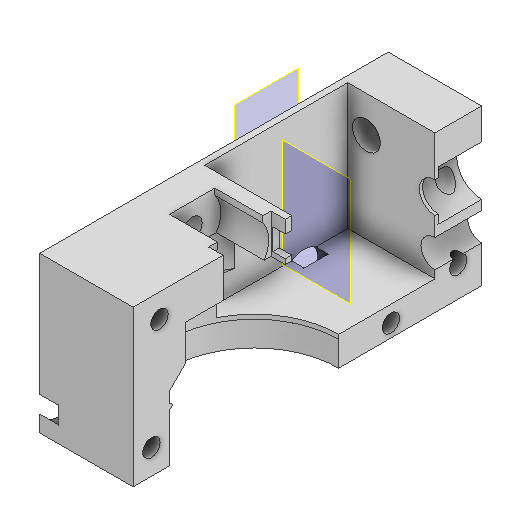
# Autodesk Inventor part: 10_SOOCT_Base_v1
Saved by Autodesk Inventor 2022 (Build 260153000, 153)
## iProperties
Created: 2023-01-02
Part Number: 10_SOOCT_Base_v1
Material: Generisch
Document SubType Name: Modeling
Designer: diederichbenedict
Density: 1 g/cm^3
Appearance: Vorgabe
Author: diederichbenedict
Autodesk Inventor part; units mm, degrees
ref_plane "YZ Plane" through (0, 0, 0) normal (1, 0, 0) x (0, 1, 0)
ref_plane "Arbeitsebene1" through (-39.7131, -1.3218, -40.6417) normal (-1, 0, 0) x (0, 0, -1)
sketch "Skizze1" plane through (-39.7131, -1.3218, -40.6417) normal (-1, 0, 0) x (0, 0, -1)
  line L0 (-10.1, 42.0592) -> (-10.1, 20.2092)
  line L1 (-10.1, 19.2092) -> (-10.1, 18.0592)
  line L2 (-37.1, 42.0592) -> (-37.1, 20.2092)
  line L3 (-37.1, 19.2092) -> (-37.1, 18.0592)
  line L4 (4, 5) -> (1, 5)
  line L5 (-37.1, 27.2) -> (-43.1, 27.2)
  line L6 (-43.1, 27.2) -> (-43.1, 3.2)
  line L7 (-43.1, 3.2) -> (-37.1, 3.2)
  line L8 (-37.1, 3.2) -> (-37.1, 27.2)
  line L9 (-7.8, 3.2) -> (0, 3.2)
  line L10 (-37.1, 3.2) -> (12.9, 3.2)
  line L11 (12.9, 3.2) -> (12.9, 27.2)
  line L12 (12.9, 27.2) -> (-37.1, 27.2)
  line L13 (-37.1, 27.2) -> (-37.1, 3.2)
  point P0 (-40.6417, -1.3218)
  point P1 (-37.1, 24.2092)
  point P2 (-7.8, 3.2)
  dimension "d0" = 0
  dimension "d2" = 6
  dimension "d3" = 50
  dimension "d21" = 24
  constraints: 28 end point, 4 horizontal, 4 parallel, 4 vertical, 2 perpendicular, 1 point on line, 12 other
  measures "d0" distance between parallel lines of L7 L9
  measures "d2" distance between parallel lines of L8 L6
  measures "d3" distance of L5.start L11.end
  measures "d21" distance between parallel lines of L12 L7
extrude "Extrusion1" add sketch "Skizze1" against normal up to surface (17 mm away)
sketch "Skizze2" plane through (-22.7131, -28.5218, 2.4583) normal (1, 0, 0) x (0, 0, -1)
  line L0 (33, 5) -> (33, 6.15)
  line L1 (33, -17.85) -> (33, 4)
  line L2 (0, 24) -> (56, 24)
  line L3 (8.5007, 24) -> (8.5007, 12.0658)
  line L4 (8.5007, 12.0658) -> (5.9, 9.4651)
  line L5 (5.9, 9.4651) -> (5.9, 7.6275)
  arc A0 (5.9, 6.8275) -> (5.9, 7.6275) centre (5.9, 7.2275) ccw
  line L6 (5.9, 6.8275) -> (5.9, -14.594)
  line L7 (56.2565, 0) -> (0.3327, 0)
  line L8 (15.7023, 20.4) -> (24.9625, 20.4029)
  line L9 (19.4614, 24) -> (19.4689, 0)
  line L10 (33, 7.9908) -> (6, 7.9908) projected
  line L11 (33, 6.9908) -> (6, 6.9908) projected
  line L12 (56, 24) -> (0, 24) projected
  line L13 (6, 7.9908) -> (6, 9.1408)
  line L14 (56, 0) -> (56, 24) projected
  line L15 (56, 24) -> (0, 24) projected
  line L16 (0, 24) -> (0, 0) projected
  line L17 (0, 0) -> (56, 0) projected
  line L18 (6, 9.1408) -> (14, 17.1408)
  point P0 (2.4583, 28.5218)
  point P1 (5.9, 0)
  point P2 (7.3142, 24)
  dimension "d10" = 5.5
  dimension "d37" = 0
  dimension "d38" = 0.1
  dimension "d39" = 0
  dimension "d40" = 0.8
  dimension "d41" = 0.3
  constraints: 24 end point, 6 point on line, 2 collinear, 2 parallel, 2 point on circle, 1 centre point, 1 coincident, 1 vertical, 3 other
  measures "d10" distance from line of L8.end L9
  measures "d37" distance between parallel lines of L12 L2
  measures "d38" distance between parallel lines of L13 L5
  measures "d39" distance between parallel lines of L6 L5
  measures "d40" distance of L5.end L6.start
  measures "d41" distance between parallel lines of L18 L4
revolve "Umdrehung1" cut sketch "Skizze2" angle 360 about axis through (-22.7131, -4.5218, -17.0031) along (0, -1, -0.0003154) contours L2 L9 L11 A0 L5 L4 L3 | L6 A0 L11 L9 L7
sketch "Skizze3" plane through (-22.7131, -28.5218, -53.5417) normal (1, 0, 0) x (0, 0, -1)
  line L0 (-38.5, 18.2) -> (-38.5, 22.2) projected
  line L1 (-34.5, 18.2) -> (-38.5, 18.2) projected
  line L2 (-34.5, 22.2) -> (-34.5, 18.2) projected
  line L3 (-38.5, 22.2) -> (-34.5, 22.2) projected
  line L4 (-34, 22.7) -> (-34, 17.7)
  line L5 (-34, 17.7) -> (-39, 17.7)
  line L6 (-39, 17.7) -> (-39, 22.7)
  line L7 (-39, 22.7) -> (-34, 22.7)
  line L8 (-47.4993, 12.0658) -> (-47.4993, 24) projected
  line L9 (-25.578, 24) -> (-25.5704, 12.0727) projected
  line L10 (-47.4993, 22.7) -> (-25.574, 22.7)
  line L11 (-25.574, 22.7) -> (-25.574, 17.7)
  line L12 (-25.574, 17.7) -> (-47.4993, 17.7)
  line L13 (-47.4993, 17.7) -> (-47.4993, 22.7)
  line L14 (-47.4993, 22.7) -> (-25.578, 22.7)
  line L15 (-25.578, 22.7) -> (-25.578, 24)
  line L16 (-25.578, 24) -> (-47.4993, 24)
  line L17 (-47.4993, 24) -> (-47.4993, 22.7)
  point P0 (-53.5417, 28.5218)
  point P1 (-47.4993, 17.7)
  point P2 (-34, 14.7092)
  point P3 (-25.5771, 22.7)
  point P4 (-34, 19.7092)
  point P5 (-34, 19.7092)
  point P6 (-34, 22.7)
  point P7 (-34, 17.7)
  point P8 (-47.4993, 24)
  point P9 (-25.578, 22.7)
  dimension "d12" = 0.5
  constraints: 24 end point, 4 parallel, 4 point on line, 2 horizontal, 2 perpendicular, 3 other
  measures "d12" distance between parallel lines of L3 L7
extrude "Extrusion2" add sketch "Skizze3" against normal through all contours L0 L3 L2 L1 | L10 L9 L12 L4 | L4 L5 L6 L7 | L7 L10 L8 L16 L9 | L6 L12 L8 L10 | L10 L11 L9
sketch "Skizze4" plane through (-22.7131, -28.5218, -53.5417) normal (1, 0, 0) x (0, 0, -1)
  line L0 (-38.5, 18.2) -> (-38.5, 22.2) projected
  line L1 (-34.5, 18.2) -> (-38.5, 18.2) projected
  line L2 (-34.5, 22.2) -> (-34.5, 18.2) projected
  line L3 (-38.5, 22.2) -> (-34.5, 22.2) projected
  line L4 (-34.45, 22.25) -> (-34.45, 18.15)
  line L5 (-34.45, 18.15) -> (-38.55, 18.15)
  line L6 (-38.55, 18.15) -> (-38.55, 22.25)
  line L7 (-38.55, 22.25) -> (-34.45, 22.25)
  line L8 (-56, 0) -> (-50.1, 0) projected
  line L9 (0, 0) -> (0, 24) projected
  line L10 (0, 24) -> (-25.578, 24) projected
  line L11 (-56, 24) -> (-56, 0) projected
  line L12 (-38.2, 22.25) -> (-34.8, 22.25)
  line L13 (-34.8, 22.25) -> (-34.8, 22.7)
  line L14 (-34.8, 22.7) -> (-38.2, 22.7)
  line L15 (-38.2, 22.7) -> (-38.2, 22.25)
  line L16 (-34.5, 18.2) -> (-34.5, 22.2)
  line L17 (-38.25, 18.15) -> (-34.75, 18.15)
  line L18 (-34.75, 18.15) -> (-34.75, 17.7)
  line L19 (-34.75, 17.7) -> (-38.25, 17.7)
  line L20 (-38.25, 17.7) -> (-38.25, 18.15)
  line L21 (-25.578, 24) -> (-25.5771, 22.7) projected
  line L22 (-25.5704, 12.0727) -> (-22.9681, 9.4737) projected
  line L23 (-22.9681, 9.4737) -> (-22.9669, 7.6361) projected
  arc A0 (-22.9669, 7.6361) -> (-22.9664, 6.8361) centre (-22.9667, 7.2361) ccw projected
  line L24 (-22.9664, 6.8361) -> (-22.9621, 0.0086) projected
  line L25 (-47.4993, 12.0658) -> (-47.4993, 17.7) projected
  line L26 (-50.1, 0) -> (-50.1, 6.8275) projected
  arc A1 (-50.1, 6.8275) -> (-50.1, 7.6275) centre (-50.1, 7.2275) ccw projected
  line L27 (-50.1, 7.6275) -> (-50.1, 9.4651) projected
  line L28 (-50.1, 9.4651) -> (-47.4993, 12.0658) projected
  line L29 (-47.4993, 17.7) -> (-25.574, 17.7) projected
  line L30 (-25.574, 17.7) -> (-25.5704, 12.0727) projected
  line L31 (-25.5771, 22.7) -> (-25.578, 22.7) projected
  line L32 (-22.9621, 0.0086) -> (-36.5311, 0) projected
  line L33 (-36.5311, 0) -> (0, 0) projected
  line L34 (-25.578, 22.7) -> (-25.578, 24) projected
  line L35 (-25.578, 24) -> (-56, 24) projected
  line L36 (-38.2, 22.7) -> (-34.8, 22.7)
  line L37 (-34.8, 22.7) -> (-34.8, 24)
  line L38 (-34.8, 24) -> (-38.2, 24)
  line L39 (-38.2, 24) -> (-38.2, 22.7)
  line L40 (-34.45, 21.95) -> (-21.9312, 21.95)
  line L41 (-21.9312, 21.95) -> (-21.9312, 18.5)
  line L42 (-21.9312, 18.5) -> (-34.45, 18.5)
  line L43 (-34.45, 18.5) -> (-34.45, 21.95)
  point P0 (-53.5417, 28.5218)
  point P1 (-43.6858, 14.7092)
  point P2 (-19.3142, 14.7092)
  point P3 (-47.4993, 22.7)
  point P4 (-34.75, 18.15)
  point P5 (-34.8059, 22.7)
  point P6 (-34.45, 18.5)
  dimension "d15" = 0.05
  dimension "d58" = 0.3
  dimension "d59" = 0.3
  dimension "d60" = 0.3
  dimension "d61" = 0.3
  dimension "d64" = 0.3
  dimension "d65" = 0.3
  constraints: 42 end point, 8 parallel, 5 point on line, 4 horizontal, 4 perpendicular, 3 other
  measures "d15" distance between parallel lines of L3 L7
  measures "d58" distance between parallel lines of L0 L15
  measures "d59" distance between parallel lines of L2 L37
  measures "d60" distance between parallel lines of L4 L18
  measures "d61" distance between parallel lines of L20 L6
  measures "d64" distance between parallel lines of L7 L40
  measures "d65" distance between parallel lines of L42 L1
extrude "Extrusion3" cut sketch "Skizze4" against normal blind 2 contours L0 L3 L2 L1 | L4 L5 L6 L7 | L40 L41 L42 L4 | L7 L15 L14 L13 | L14 L39 L35 L37 | L18 L19 L20 L5
sketch "Skizze5" plane through (-39.7131, -28.5218, -53.5417) normal (0, 0, -1) x (-1, 0, 0)
  arc A0 (-8, 26.2) -> (-9, 27.2) centre (-9, 26.2) ccw projected
  line L0 (-25, 27.2) -> (-9, 27.2) projected
  arc A1 (-25, 27.2) -> (-26, 26.2) centre (-25, 26.2) ccw projected
  line L1 (-26, 10.2) -> (-26, 26.2) projected
  arc A2 (-26, 10.2) -> (-25, 9.2) centre (-25, 10.2) ccw projected
  line L2 (-9, 9.2) -> (-25, 9.2) projected
  arc A3 (-9, 9.2) -> (-8, 10.2) centre (-9, 10.2) ccw projected
  line L3 (-8, 26.2) -> (-8, 10.2) projected
  circle A4 centre (-17, 18.2) radius 5.8 projected
  arc A5 (-9, 8.2) -> (-7, 10.2) centre (-9, 10.2) ccw
  line L4 (-9, 8.2) -> (-25, 8.2)
  arc A6 (-27, 10.2) -> (-25, 8.2) centre (-25, 10.2) ccw
  line L5 (-27, 10.2) -> (-27, 26.2)
  arc A7 (-25, 28.2) -> (-27, 26.2) centre (-25, 26.2) ccw
  line L6 (-25, 28.2) -> (-9, 28.2)
  arc A8 (-7, 26.2) -> (-9, 28.2) centre (-9, 26.2) ccw
  line L7 (-7, 26.2) -> (-7, 10.2)
  line L8 (-31, 32.2) -> (-3, 32.2)
  line L9 (-3, 32.2) -> (-3, 4.2)
  line L10 (-3, 4.2) -> (-31, 4.2)
  line L11 (-31, 4.2) -> (-31, 32.2)
  line L12 (-31, 32.2) -> (-3, 4.2) construction
  line L13 (-3, 32.2) -> (-31, 4.2) construction
  point P0 (-39.7131, 28.5218)
  dimension "d18" = 1
  dimension "d27" = 28
  dimension "d28" = 28
  constraints: 20 end point, 8 point on circle, 4 centre point, 2 midpoint, 2 parallel, 1 horizontal, 1 perpendicular, 7 other
  measures "d18" distance between parallel lines of L3 L7
  measures "d27" distance of L9.end L10.end
  measures "d28" distance of L8.end L9.end
extrude "Extrusion4" cut sketch "Skizze5" against normal blind 23.5 contours L3 A3 L2 A2 L1 A1 L0 A0 | A4 | L4 A6 L5 A7 L6 A8 L7 A5
sketch "Skizze6" plane through (-39.7131, -28.5218, -53.5417) normal (0, 0, -1) x (-1, 0, 0)
  line L0 (-9, 8.2) -> (-17, 8.2) projected
  line L1 (-17, 0) -> (-17, 8.2) projected
  line L2 (0, 0) -> (-17, 0) projected
  line L3 (0, 24) -> (0, 0) projected
  line L4 (0, 24) -> (-7, 24) projected
  line L5 (-7, 24) -> (-7, 10.2) projected
  arc A0 (-9, 8.2) -> (-7, 10.2) centre (-9, 10.2) ccw projected
  line L6 (-17, 8.2) -> (-17, 12.0727) projected
  line L7 (-17, 8.2) -> (-7, 8.2)
  line L8 (-7, 8.2) -> (-7, 24)
  line L9 (-7, 24) -> (-17, 24)
  line L10 (-17, 24) -> (-17, 8.2)
  circle A1 centre (-17, 18.2) radius 4 projected
  circle A2 centre (-17, 15.0113) radius 4
  point P0 (-39.7131, 28.5218)
  point P1 (-17, 22.2)
  point P2 (-17, 14.2)
  point P3 (-17, 19.0113)
  point P4 (-17, 11.0113)
  constraints: 8 end point, 2 parallel, 1 centre point, 1 horizontal, 1 perpendicular, 2 other
ref_plane "Arbeitsebene2" through (-26.7131, -14.3218, -41.6417) normal (0, 0, 1) x (1, 0, 0)
ref_plane "Arbeitsebene3" through (-26.7131, -14.3218, -44.6417) normal (0, 0, -1) x (0, 1, 0)
extrude "Extrusion5" add sketch "Skizze6" against normal blind 8 contours L0 L6 A2 A1 L10 L9 L5 A0 | A1 A2 L10 picked at (-16.3965, 20.005)
sketch "Skizze7" plane through (-32.7131, -4.5218, -45.5417) normal (0, 0, 1) x (1, 0, 0)
  circle A0 centre (10, -5.8) radius 4
  line L0 (10, 0) -> (10, -24) projected
  line L1 (10, -9.8) -> (10, -1.8)
  circle A1 centre (10, -5.8) radius 3
  circle A2 centre (10, -8.9887) radius 4 projected
  point P0 (32.7131, 4.5218)
  point P1 (10, -8.8)
  point P2 (10, -2.8)
  dimension "d24" = 1
  constraints: 2 centre point, 2 end point, 1 point on circle
  measures "d24" radial gap between concentric circles of A0 A1
extrude "Extrusion6" add sketch "Skizze7" against normal blind 0.5 contours L0 A1 A2 A0 | A2 A1 L0 A0 picked at (9.6732, -2.174) picked at (9.6932, -9.4309)
ref_plane "Arbeitsebene4" through (-39.7131, -28.5218, -32.0417) normal (0, 0, -1) x (-1, 0, 0)
sketch "Skizze8" plane through (-39.7131, -28.5218, -32.0417) normal (0, 0, -1) x (-1, 0, 0)
  circle A0 centre (-17, 18.2) radius 4 projected
  line L0 (-3, 3.7) -> (-31, 3.7)
  line L1 (-31, 3.7) -> (-31, 32.7)
  line L2 (-31, 32.7) -> (-3, 32.7)
  line L3 (-3, 32.7) -> (-3, 3.7)
  line L4 (-17, 22.2) -> (-17, 18.2) projected
  line L5 (-3, 3.7) -> (-31, 32.7) construction
  line L6 (-31, 3.7) -> (-3, 32.7) construction
  point P0 (-39.7131, 28.5218)
  dimension "d30" = 28
  dimension "d31" = 29
  constraints: 12 end point, 2 midpoint, 2 parallel, 1 horizontal, 1 perpendicular, 1 vertical alignment
  measures "d30" distance of L1.end L2.end
  measures "d31" distance of L0.end L1.end
extrude "Extrusion7" cut sketch "Skizze8" along normal blind 14 and the other way blind 9 contours A0 | L0 L1 L2 L3
sketch "Skizze9" plane through (-39.7131, -28.5218, -53.5417) normal (0, 0, -1) x (-1, 0, 0)
  circle A0 centre (-17, 7.2) radius 2.2504 projected
  circle A1 centre (-6, 18.2) radius 2.2504 projected
  point P0 (-39.7131, 28.5218)
extrude "Extrusion8" cut sketch "Skizze9" against normal blind 14
sketch "Skizze10" plane through (-39.7131, -28.5218, -53.5417) normal (0, -1, 0) x (1, 0, 0)
  line L0 (8.5019, 6.0924) -> (3.4981, 6.0924) projected
  line L1 (17, 56) -> (17, 50.1) projected
  line L2 (0, 56) -> (17, 56) projected
  line L3 (0, 0) -> (0, 56) projected
  line L4 (0, 0) -> (17, 0) projected
  line L5 (17, 36.5311) -> (17, 0) projected
  line L6 (17, 50.1) -> (17, 36.5311) projected
  ellipse E0 centre (17, 36.5311) end of major axis (30.5689, 36.5311) minor radius 13.5689 (17, 50.1) -> (17, 22.9621) ccw projected
  point P0 (39.7131, 53.5417)
  constraints: 1 other
extrude "Extrusion9" cut sketch "Skizze10" against normal blind 3 contours L6 L5 E0
sketch "Skizze11" plane through (-39.7131, -28.5218, -53.5417) normal (0, -1, 0) x (1, 0, 0)
  circle A0 centre (17, 36.5) radius 13.5 projected
  ellipse E0 centre (17, 36.5311) end of major axis (30.5689, 36.5311) minor radius 13.5689 (17, 50.1) -> (17, 22.9621) ccw projected
  line L0 (17, 56) -> (17, 50.1) projected
  line L1 (0, 56) -> (17, 56) projected
  line L2 (0, 0) -> (0, 56) projected
  line L3 (0, 0) -> (17, 0) projected
  line L4 (17, 22.9621) -> (17, 0) projected
  point P0 (39.7131, 53.5417)
  constraints: 1 other
extrude "Extrusion10" add sketch "Skizze11" along normal blind 3 contours E0 L4 L3 L2 L1 L0
sketch "Skizze12" plane through (-39.7131, -1.3218, -40.6417) normal (-1, 0, 0) x (0, 0, 1)
  circle A0 centre (40.15, -24.2) radius 1.29
  circle A1 centre (38.86, -7) radius 1.4
  circle A2 centre (-9.15, -23.4127) radius 1.4
  circle A3 centre (1.6677, -26.1156) radius 1.4
  circle A4 centre (-10.55, -14.0018) radius 1.4
  line L0 (-12.9, -11.2504) -> (-5.4, -11.2504) projected
  line L1 (-12.9, -22.2504) -> (-5.4, -22.2504) projected
  line L2 (-12.9, -6.7496) -> (-5.4, -6.7496) projected
  point P0 (40.6417, 1.3218)
  dimension "d46" = 2.58
  dimension "d47" = 2.8
  dimension "d48" = 2.8
  dimension "d49" = 2.8
  dimension "d50" = 2.8
  constraints: 5 centre point
  measures "d46" diameter of A0
  measures "d47" diameter of A1
  measures "d48" diameter of A2
  measures "d49" diameter of A3
  measures "d50" diameter of A4
hole "Bohrung1" at (-39.7131, -25.5218, -0.4917) at (-39.7131, -8.3218, -1.7817) at (-39.7131, -27.4374, -38.974) at (-39.7131, -24.7346, -49.7917) at (-39.7131, -15.3236, -51.1917) direction (1, 0, 0) diameter 2.8 end through all counterbore diameter 6.5 counterbore depth 5
sketch "Skizze13" plane through (-39.7131, -1.3218, -40.6417) normal (-1, 0, 0) x (0, 0, 1)
  line L0 (37.2, -30.2) -> (43.1, -30.2) projected
  line L1 (43.1, -30.2) -> (-14.489, -30.2)
  line L2 (-14.489, -30.2) -> (-14.489, -1.9274)
  line L3 (-14.489, -1.9274) -> (43.1, -1.9274)
  line L4 (43.1, -1.9274) -> (43.1, -30.2)
  point P0 (40.6417, 1.3218)
  point P1 (37.2, -30.2)
  constraints: 8 end point, 2 parallel, 1 horizontal, 1 perpendicular
extrude "Extrusion11" cut sketch "Skizze13" against normal blind 2
sketch "Skizze14" plane through (-39.7131, -28.5218, -46.0417) normal (0, 0, 1) x (1, 0, 0)
  arc A0 (17, 19.0113) -> (17, 11.0113) centre (17, 15.0113) ccw projected
  circle A1 centre (17, 15.0113) radius 2.5
  line L0 (17, 11.0113) -> (17, 9.4504) projected
  line L1 (17, 11.0113) -> (17, 19.0113)
  point P0 (39.7131, 28.5218)
  point P1 (17, 12.5113)
  point P2 (17, 17.5113)
  dimension "d68" = 5
  constraints: 2 end point, 1 centre point, 1 coincident, 1 collinear
  measures "d68" diameter of A1
extrude "Extrusion12" add sketch "Skizze14" against normal blind 0.5 contours L1 A1 A0
sketch "Skizze15" plane through (-37.7131, -1.3218, -40.6417) normal (-1, 0, 0) x (0, 0, 1)
  circle A0 centre (1.6677, -26.1156) radius 3.25 projected
  circle A1 centre (38.86, -7) radius 3.25 projected
  circle A2 centre (-9.15, -23.4127) radius 3.25 projected
  arc A3 (43.1, -22.8362) -> (43.1, -25.5638) centre (40.15, -24.2) ccw projected
  line L0 (43.1, -3.2) -> (43.1, -22.8362) projected
  line L1 (-12.9, -3.2) -> (43.1, -3.2) projected
  line L2 (-12.9, -11.7568) -> (-12.9, -3.2) projected
  arc A4 (-12.9, -16.2468) -> (-12.9, -11.7568) centre (-10.55, -14.0018) ccw projected
  line L3 (-12.9, -30.2) -> (-12.9, -16.2468) projected
  line L4 (43.1, -30.2) -> (-12.9, -30.2) projected
  line L5 (43.1, -25.5638) -> (43.1, -30.2) projected
  line L6 (43.1, -3.2) -> (43.1, -30.2) projected
  line L7 (-12.9, -30.2) -> (43.1, -30.2)
  line L8 (43.1, -30.2) -> (43.1, -28.2)
  line L9 (43.1, -28.2) -> (-12.9, -28.2)
  line L10 (-12.9, -28.2) -> (-12.9, -30.2)
  point P0 (40.6417, 1.3218)
  dimension "d71" = 2
  constraints: 8 end point, 2 parallel, 1 horizontal, 1 perpendicular, 1 point on line
  measures "d71" distance of L8.end L7.end
extrude "Extrusion13" cut sketch "Skizze15" against normal through all contours L9 A0 | A0 L9 L5 L4 L3 picked at (1.0341, -28.384)
sketch "Skizze16" plane through (-22.7131, -20.8943, -3.4417) normal (1, 0, 0) x (0, 0, -1)
  circle A0 centre (13.6, 12.5725) radius 4.6
  line L0 (50.1, 16.3725) -> (-5.9, 16.3725) projected
  line L1 (9.9503, 16.3725) -> (9.9503, 15.3725)
  line L2 (9.9503, 16.3725) -> (10.9503, 16.3725) construction
  line L3 (17.2497, 16.3725) -> (17.2497, 15.3725)
  line L4 (11.55, 14.6225) -> (15.65, 10.5225)
  line L5 (15.65, 10.5225) -> (15.65, 14.6225)
  line L6 (15.65, 14.6225) -> (11.55, 10.5225)
  point P0 (-3.4417, 20.8943)
  point P1 (16.1923, 16.3725)
  point P2 (11.0077, 16.3725)
  dimension "d74" = 9.2
  dimension "d80" = 90
  dimension "d81" = 1
  dimension "d82" = 1
  constraints: 12 end point, 3 midpoint, 2 perpendicular, 2 point on circle, 2 point on line, 2 vertical, 1 centre point, 1 horizontal
  measures "d74" diameter of A0
  measures "d80" angle of L1 L2
  measures "d81" distance of L1.end L1.start
  measures "d82" distance from line of L3.end L0
extrude "Extrusion14" cut sketch "Skizze16" against normal blind 10 contours A0 L0 | A0 L0 L3 | L1 L0 A0 | L0 A0 | L6 L5 L4
sketch "Skizze18" plane through (-22.7131, -20.8943, -3.4417) normal (1, 0, 0) x (0, 0, -1)
  line L0 (9.9503, 15.3725) -> (9.9503, 16.3725) projected
  line L1 (9.9503, 16.3725) -> (-5.9, 16.3725) projected
  line L2 (-5.9, 16.3725) -> (-5.9, -8.6275) projected
  line L3 (-5.9, -8.6275) -> (0, -8.6275) projected
  line L4 (0, -4.6275) -> (0, -8.6275) projected
  line L5 (0, -4.6275) -> (0, -0.8) projected
  arc A0 (0, -0.8) -> (0, 0) centre (0, -0.4) ccw projected
  line L6 (0, 0) -> (0, 1.8376) projected
  line L7 (0, 1.8376) -> (2.6007, 4.4383) projected
  line L8 (2.6007, 4.4383) -> (2.6007, 10.0725) projected
  line L9 (2.6007, 10.0725) -> (9.7387, 10.0725) projected
  arc A1 (9.9503, 15.3725) -> (9.7387, 10.0725) centre (13.6, 12.5725) ccw projected
  circle A2 centre (-2.95, -4.6275) radius 1.4 projected
  circle A3 centre (-1.66, 12.5725) radius 1.4 projected
  arc A4 (8.9719, 11.9725) -> (10.3013, 10.0882) centre (10.9719, 11.9725) ccw projected
  arc A5 (11.9719, 16.3512) -> (10.3013, 10.0882) centre (13.5632, 12.5725) ccw projected
  line L10 (11.9719, 16.6725) -> (11.9719, 16.3512) projected
  line L11 (8.9719, 16.6725) -> (11.9719, 16.6725) projected
  line L12 (8.9719, 11.9725) -> (8.9719, 16.6725) projected
  line L13 (18.5632, 7.5725) -> (8.5632, 7.5725)
  line L14 (8.5632, 7.5725) -> (8.5632, 17.5725)
  line L15 (8.5632, 17.5725) -> (18.5632, 17.5725)
  line L16 (18.5632, 17.5725) -> (18.5632, 7.5725)
  line L17 (18.5632, 7.5725) -> (8.5632, 17.5725) construction
  line L18 (8.5632, 7.5725) -> (18.5632, 17.5725) construction
  point P0 (-3.4417, 20.8943)
  point P1 (9.36, 10.7885)
  point P2 (8.5632, 10.0725)
  point P3 (8.5632, 16.3725)
  point P4 (8.9719, 16.3725)
  dimension "d83" = 10
  dimension "d84" = 10
  constraints: 12 end point, 2 midpoint, 2 parallel, 1 coincident, 1 horizontal, 1 perpendicular
  measures "d83" distance of L14.end L15.end
  measures "d84" distance of L13.end L14.end
extrude "Extrusion16" cut sketch "Skizze18" against normal blind 2.3 contours A1 A4 L12 L1 L0 | L0 L1 L12 L11 L10 A5 A4 A1 | A4 A5 L10 L11 L12 L1 L14 L15 L16 L13 L9 A1 | A1 L9 L14 L1 L12 A4
sketch "Skizze19" plane through (-37.7131, -1.3218, -40.6417) normal (-1, 0, 0) x (0, 0, 1)
  circle A0 centre (23.6, -7) radius 1.5 projected
  circle A1 centre (23.6, -7) radius 1.6
  point P0 (40.6417, 1.3218)
  dimension "d87" = 3.2
  constraints: 1 centre point, 1 coincident
  measures "d87" diameter of A1
extrude "Extrusion17" cut sketch "Skizze19" against normal through all contours A0 | A1
equation "\"d59\" = d58"
equation "\"d60\" = d58"
equation "\"d61\" = d58"
equation "\"d64\" = d58"
equation "\"d65\" = d58"
